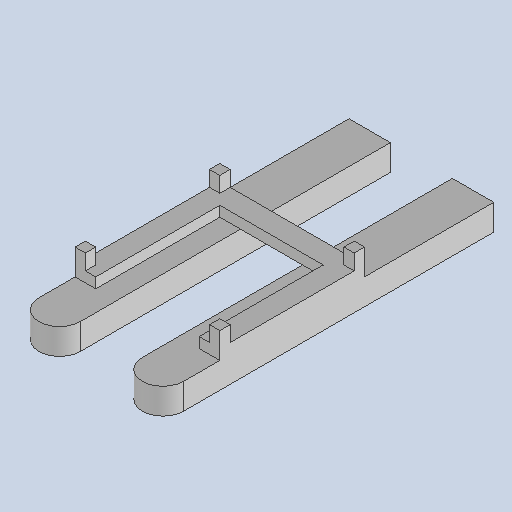
# Autodesk Inventor part: pallet jack dummy_1200
Saved by Autodesk Inventor 2026.2 (Build 302298000, 298)
## iProperties
Created: 2025-12-18
Part Number: pallet jack dummy_1200
Material: Generic
Document SubType Name: Modeling
Designer: admin
Density: 1 g/cm^3
Appearance: Default
Author: admin
Autodesk Inventor part; units mm, degrees
ref_plane "YZ Plane" through (0, 0, 0) normal (1, 0, 0) x (0, 1, 0)
ref_plane "XZ Plane" through (0, 0, 0) normal (0, 1, 0) x (-1, 0, 0)
ref_plane "XY Plane" through (0, 0, 0) normal (0, 0, 1) x (1, 0, 0)
sketch "Sketch1" plane through (0, 0, 0) normal (0, 0, 1) x (1, 0, 0)
  line L0 (280, 0) -> (280, -1200)
  arc A0 (120, -1200) -> (280, -1200) centre (200, -1200) ccw
  line L1 (120, -1200) -> (120, 0)
  line L2 (-120, 0) -> (-120, -1200)
  arc A1 (-280, -1200) -> (-120, -1200) centre (-200, -1200) ccw
  line L3 (-280, -1200) -> (-280, 0)
  line L4 (280, 0) -> (-280, 0)
  line L5 (0, 0) -> (0, -1425.5319) construction
  dimension "d0" = 160
  dimension "d1" = 560
  dimension "d2" = 1200
  constraints: 12 end point, 4 point on circle, 4 tangent, 3 vertical, 2 centre point, 2 parallel, 1 equal radius, 1 horizontal, 1 midpoint, 1 point on line, 1 other
  measures "d0" distance between parallel lines of L1 L0
  measures "d1" distance between parallel lines of L3 L0
  measures "d2" distance from line of L4 A1.centre
extrude "Extrusion1" add sketch "Sketch1" along normal blind 100
sketch "Sketch2" plane through (0, 0, 100) normal (0, 0, 1) x (1, 0, 0)
  arc A0 (-280, -1200) -> (-120, -1200) centre (-200, -1200) ccw projected
  line L0 (-120, -1200) -> (-120, 0) projected
  line L1 (-120, 0) -> (-280, 0) projected
  line L2 (-280, 0) -> (-280, -1200) projected
  line L3 (280, 0) -> (120, 0) projected
  line L4 (120, 0) -> (120, -1200) projected
  arc A1 (120, -1200) -> (280, -1200) centre (200, -1200) ccw projected
  line L5 (280, -1200) -> (280, 0) projected
  line L6 (-280, -1060) -> (-200, -1060)
  line L7 (-200, -1060) -> (-200, -500)
  line L8 (-200, -500) -> (-280, -500)
  line L9 (-280, -500) -> (-280, -1060)
  line L10 (200, -1060) -> (280, -1060)
  line L11 (280, -1060) -> (280, -500)
  line L12 (280, -500) -> (200, -500)
  line L13 (200, -500) -> (200, -1060)
  line L14 (-200, -500) -> (200, -500)
  line L15 (200, -500) -> (200, -580)
  line L16 (200, -580) -> (-200, -580)
  line L17 (-200, -580) -> (-200, -500)
  line L18 (-280, 0) -> (-280, -1200) projected
  line L19 (280, -1200) -> (280, 0) projected
  point P0 (0, 0)
  point P1 (-200, -580)
  dimension "d5" = 80
  dimension "d6" = 560
  dimension "d7" = 560
  dimension "d8" = 400
  dimension "d9" = 500
  constraints: 24 end point, 6 parallel, 3 horizontal, 3 perpendicular, 3 point on line, 2 collinear, 2 equal length
  measures "d5" distance of L6.start L6.end
  measures "d6" distance between parallel lines of L5 L2
  measures "d7" distance of L6.end L7.end
  measures "d8" distance of L15.end L16.end
  measures "d9" distance between parallel lines of L1 L8
extrude "Extrusion2" add sketch "Sketch2" along normal blind 40 contours L2 L8 L7 L6 | L16 L7 L14 L0 | L0 L14 L4 L16 | L4 L14 L13 L16 | L13 L12 L5 L10
sketch "Sketch3" plane through (0, 0, 140) normal (0, 0, 1) x (1, 0, 0)
  line L0 (-280, -500) -> (-280, -1060) projected
  line L1 (-280, -1060) -> (-200, -1060) projected
  line L2 (-200, -1060) -> (-200, -580) projected
  line L3 (-200, -580) -> (200, -580) projected
  line L4 (200, -580) -> (200, -1060) projected
  line L5 (200, -1060) -> (280, -1060) projected
  line L6 (280, -1060) -> (280, -500) projected
  line L7 (280, -500) -> (-280, -500) projected
  line L8 (-280, -1060) -> (-240, -1060)
  line L9 (-240, -1060) -> (-240, -1020)
  line L10 (-240, -1020) -> (-280, -1020)
  line L11 (-280, -1020) -> (-280, -1060)
  line L12 (-280, -500) -> (-240, -500)
  line L13 (-240, -500) -> (-240, -540)
  line L14 (-240, -540) -> (-280, -540)
  line L15 (-280, -540) -> (-280, -500)
  line L16 (280, -500) -> (240, -500)
  line L17 (240, -500) -> (240, -540)
  line L18 (240, -540) -> (280, -540)
  line L19 (280, -540) -> (280, -500)
  line L20 (280, -1060) -> (240, -1060)
  line L21 (240, -1060) -> (240, -1020)
  line L22 (240, -1020) -> (280, -1020)
  line L23 (280, -1020) -> (280, -1060)
  point P0 (0, 0)
  dimension "d12" = 40
  constraints: 32 end point, 8 parallel, 6 equal length, 4 horizontal, 4 perpendicular, 1 point on line
  measures "d12" distance of L10.end L9.end
extrude "Extrusion3" add sketch "Sketch3" along normal blind 60 contours L7 L13 L14 L0 | L10 L9 L1 L0 | L7 L6 L18 L17 | L6 L5 L21 L22
equation "\"d7\" = d6"
body "Solid1"
